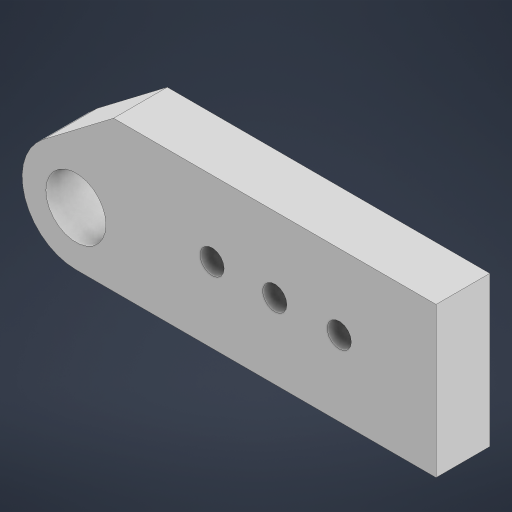
# Autodesk Inventor part: Slide_Climb_Mounts
Saved by Autodesk Inventor 2023 (Build 270158000, 158)
## iProperties
Created: 2024-02-26
Part Number: Slide_Climb_Mounts
Material: Generic
Document SubType Name: Modeling
Designer: kelle
Density: 1 g/cm^3
Appearance: Default
Author: kelle
Autodesk Inventor part; units mm, degrees
ref_plane "YZ Plane" through (0, 0, 0) normal (1, 0, 0) x (0, 1, 0)
ref_plane "XZ Plane" through (0, 0, 0) normal (0, 1, 0) x (-1, 0, 0)
ref_plane "XY Plane" through (0, 0, 0) normal (0, 0, 1) x (1, 0, 0)
sketch "Sketch1" plane through (0, 0, 0) normal (0, 0, 1) x (1, 0, 0)
  line L0 (38.1, -17.7165) -> (-38.1, -17.7165)
  line L1 (-38.1, -17.7165) -> (-38.1, 17.7165)
  line L2 (-38.1, 17.7165) -> (38.1, 17.7165)
  line L3 (38.1, 17.7165) -> (38.1, -17.7165)
  line L4 (38.1, -17.7165) -> (-38.1, 17.7165) construction
  line L5 (-38.1, -17.7165) -> (38.1, 17.7165) construction
  circle A0 centre (-14.825, 0) radius 2.85
  circle A1 centre (0, 0) radius 2.85
  circle A2 centre (15.225, 0) radius 2.85
  circle A3 centre (-46.99, -5.0165) radius 7.1
  circle A4 centre (-46.99, -5.0165) radius 12.7
  line L6 (-38.1, -17.7165) -> (-46.99, -17.7165)
  line L7 (-38.1, 17.7165) -> (-54.6842, 5.0874)
  dimension "d0" = 76.2
  dimension "d1" = 35.433
  dimension "d2" = 5.7
  dimension "d3" = 14.825
  dimension "d4" = 5.7
  dimension "d5" = 5.7
  dimension "d6" = 15.225
  dimension "d7" = 14.2
  dimension "d8" = 8.89
  dimension "d9" = 12.7
  dimension "d10" = 25.4
  constraints: 16 end point, 5 centre point, 2 coincident, 2 midpoint, 2 parallel, 2 point on circle, 1 horizontal, 1 perpendicular, 1 point on line, 1 tangent
  measures "d0" distance of L1.end L2.end
  measures "d1" distance of L0.end L1.end
  measures "d2" diameter of A0
  measures "d3" distance of point (0, 0) A0.centre
  measures "d4" diameter of A1
  measures "d5" diameter of A2
  measures "d6" distance of A1.centre A2.centre
  measures "d7" diameter of A3
  measures "d8" distance from line of L1 A3.centre
  measures "d9" distance from line of L0 A3.centre
  measures "d10" diameter of A4
extrude "Extrusion1" add sketch "Sketch1" along normal blind 12.7
extrude "Extrusion2" add sketch "Sketch1" along normal blind 3.7 contours A0 | A1 | A2
body "Solid1"
